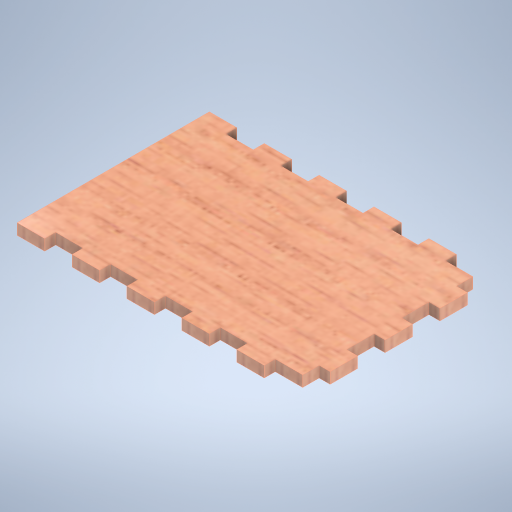
# Autodesk Inventor part: ER_lipo_back_1
Saved by Autodesk Inventor 2023 (Build 270158000, 158)
## iProperties
Created: 2023-03-05
Part Number: ER_lipo_back_1
Material: 木材 (オーク)
Document SubType Name: Modeling
Designer: mkhr7
Density: 0.76 g/cm^3
Appearance: ホワイト オーク材 - ナチュラル 標準の光沢
Author: mkhr7
Autodesk Inventor part; units mm, degrees
ref_plane "YZ Plane" through (0, 0, 0) normal (1, 0, 0) x (0, 1, 0)
ref_plane "XZ Plane" through (0, 0, 0) normal (0, 1, 0) x (-1, 0, 0)
ref_plane "XY Plane" through (0, 0, 0) normal (0, 0, 1) x (1, 0, 0)
sketch "スケッチ1" plane through (0, 0, 0) normal (0, 1, 0) x (-1, 0, 0)
  line L0 (0, 0) -> (100, 0)
  line L1 (100, 0) -> (100, -70)
  line L2 (100, -70) -> (0, -70)
  line L3 (0, -70) -> (0, 0)
  line L4 (0, -10) -> (-4, -10)
  line L5 (-4, -10) -> (-4, -20)
  line L6 (-4, -20) -> (0, -20)
  line L7 (0, -20) -> (0, -10)
  line L8 (0, -30) -> (-4, -30)
  line L9 (-4, -30) -> (-4, -40)
  line L10 (-4, -40) -> (0, -40)
  line L11 (0, -50) -> (-4, -50)
  line L12 (-4, -50) -> (-4, -60)
  line L13 (-4, -60) -> (0, -60)
  line L14 (0, 0) -> (10, 0)
  line L15 (10, 0) -> (10, -4)
  line L16 (10, -4) -> (0, -4)
  line L17 (0, -4) -> (0, 0)
  line L18 (0, -70) -> (10, -70)
  line L19 (10, -70) -> (10, -66)
  line L20 (10, -66) -> (0, -66)
  line L21 (0, -66) -> (0, -70)
  line L22 (30, 0) -> (20, 0)
  line L23 (20, 0) -> (20, -4)
  line L24 (20, -4) -> (30, -4)
  line L25 (30, -4) -> (30, 0)
  line L26 (30, -70) -> (20, -70)
  line L27 (20, -70) -> (20, -66)
  line L28 (20, -66) -> (30, -66)
  line L29 (30, -66) -> (30, -70)
  line L30 (50, -4) -> (50, 0)
  line L31 (40, -4) -> (50, -4)
  line L32 (40, 0) -> (40, -4)
  line L33 (50, -66) -> (50, -70)
  line L34 (40, -66) -> (50, -66)
  line L35 (40, -70) -> (40, -66)
  line L36 (70, -4) -> (70, 0)
  line L37 (60, -4) -> (70, -4)
  line L38 (60, 0) -> (60, -4)
  line L39 (70, -66) -> (70, -70)
  line L40 (60, -66) -> (70, -66)
  line L41 (60, -70) -> (60, -66)
  line L42 (90, -4) -> (90, 0)
  line L43 (80, -4) -> (90, -4)
  line L44 (80, 0) -> (80, -4)
  line L45 (90, -66) -> (90, -70)
  line L46 (80, -66) -> (90, -66)
  line L47 (80, -70) -> (80, -66)
  point P0 (20, -2)
  point P1 (40, -2)
  point P2 (60, -2)
  point P3 (80, -2)
  point P4 (0, -20)
  point P5 (0, -40)
  point P6 (0, -60)
  dimension "d0" = 100
  dimension "d1" = 70
  dimension "d2" = 4
  dimension "d3" = 10
  dimension "d4" = 10
  dimension "d7" = 20
  dimension "d12" = 10
  dimension "d13" = 4
  dimension "d14" = 10
  dimension "d15" = 4
  dimension "d16" = 10
  dimension "d17" = 10
  dimension "d18" = 10
  dimension "d21" = 20
  constraints: 96 end point, 12 parallel, 7 horizontal, 7 point on line, 6 perpendicular, 1 midpoint, 1 vertical, 59 other
  measures "d0" distance of L1.end L2.end
  measures "d1" distance of L0.end L1.end
  measures "d2" distance of L6.end L5.end
  measures "d3" distance of L5.end L4.end
  measures "d4" distance from line of L0.start L4
  measures "d7" distance of L4.start L8.start
  measures "d12" distance of L15.end L16.end
  measures "d13" distance of L14.end L15.end
  measures "d14" distance of L20.end L19.end
  measures "d15" distance of L19.end L18.end
  measures "d16" distance of L24.end L23.end
  measures "d17" distance of L27.end L28.end
  measures "d18" distance from line of point (20, -2) L15
  measures "d21" distance of L24.end L30.start
extrude "押し出し1" add sketch "スケッチ1" along normal blind 4 contours L0 L23 L24 L25 L32 L31 L30 L38 L37 L36 L44 L43 L42 L1 L2 L45 L46 L47 L39 L40 L41 L33 L34 L35 L29 L28 L27 L19 L20 L3 L16 L15 | L3 L6 L5 L4 | L3 L10 L9 L8 | L3 L13 L12 L11
